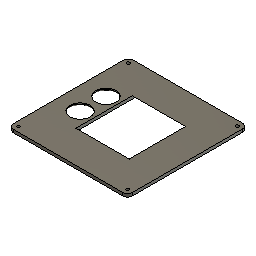
Case_Bottom (Autodesk Fusion 360 design; units mm, degrees)
part number: 2026-02-15-14-31-26-790
Autodesk Fusion 360 part; units mm, degrees
(part 1 of 2)
sketch "Sketch1" plane through (0, 0, 0) normal (0, 1, 0) x (1, 0, 0)
  line L0 (0, 0) -> (98.4, 0)
  line L1 (98.4, 0) -> (98.4, 99.18)
  line L2 (98.4, 99.18) -> (0, 99.18)
  line L3 (0, 99.18) -> (0, 0)
  line L4 (-10, 109.18) -> (108.4, 109.18)
  line L5 (108.4, 109.18) -> (108.4, -10)
  line L6 (108.4, -10) -> (-10, -10)
  line L7 (-10, -10) -> (-10, 109.18)
  circle A0 centre (-5, 104.18) radius 1.45
  circle A1 centre (103.4, 104.18) radius 1.45
  circle A2 centre (-5, -5) radius 1.45
  circle A3 centre (103.4, -5) radius 1.45
  dimension "d1" = 98.4
  dimension "d2" = 99.18
  dimension "d3" = 10
  dimension "d4" = 10
  dimension "d5" = 10
  dimension "d6" = 10
  dimension "d7" = 2.9
  dimension "d8" = 2.9
  dimension "d9" = 2.9
  dimension "d10" = 2.9
  dimension "d11" = 5
  dimension "d12" = 5
  dimension "d13" = 5
  dimension "d14" = 5
  dimension "d15" = 5
  dimension "d16" = 5
  dimension "d17" = 5
  dimension "d18" = 5
  constraint horizontal L0
  constraint vertical L1
  constraint horizontal L2
  constraint vertical L3
  constraint coincident L0.start L3.end
  constraint horizontal L4
  constraint vertical L5
  constraint horizontal L6
  constraint vertical L7
  measures "d1" distance of L0.start L0.end
  measures "d2" distance of L0.start L2.end
  measures "d3" distance of L1 L5
  measures "d4" distance of L3 L7
  measures "d5" distance of L0 L6
  measures "d6" distance of L2 L4
  measures "d7" diameter of A0
  measures "d8" diameter of A1
  measures "d9" diameter of A2
  measures "d10" diameter of A3
  measures "d11" distance of L6 A2.centre
  measures "d12" distance of L7 A2.centre
  measures "d13" distance of L6 A3.centre
  measures "d14" distance of L5 A3.centre
  measures "d15" distance of L4 A1.centre
  measures "d16" distance of L5 A1.centre
  measures "d17" distance of L4 A0.centre
  measures "d18" distance of L7 A0.centre
extrude "Extrude1" add sketch "Sketch1" along normal blind 3 contours L0 L1 L2 L3 | L4 L5 L6 L7 makes body 1
extrude "Extrude2" add sketch "Sketch1" along normal blind 13 bodies 1
sketch "plate-2026-02-16T06_39_50.723Z" plane through (0, 13, 0) normal (0, 1, 0) x (1, 0, 0)
  line L0 (38.525, 61.075) -> (51.525, 61.075)
  line L1 (38.525, 47.075) -> (51.525, 47.075)
  line L2 (38.025, 60.575) -> (38.025, 47.575)
  line L3 (52.025, 60.575) -> (52.025, 47.575)
  arc A0 (38.525, 61.075) -> (38.025, 60.575) centre (38.525, 60.575) ccw
  arc A1 (52.025, 60.575) -> (51.525, 61.075) centre (51.525, 60.575) ccw
  arc A2 (38.025, 47.575) -> (38.525, 47.075) centre (38.525, 47.575) ccw
  arc A3 (51.525, 47.075) -> (52.025, 47.575) centre (51.525, 47.575) ccw
  line L4 (57.575, 61.075) -> (70.575, 61.075)
  line L5 (57.575, 47.075) -> (70.575, 47.075)
  line L6 (57.075, 60.575) -> (57.075, 47.575)
  line L7 (71.075, 60.575) -> (71.075, 47.575)
  arc A4 (57.575, 61.075) -> (57.075, 60.575) centre (57.575, 60.575) ccw
  arc A5 (71.075, 60.575) -> (70.575, 61.075) centre (70.575, 60.575) ccw
  arc A6 (57.075, 47.575) -> (57.575, 47.075) centre (57.575, 47.575) ccw
  arc A7 (70.575, 47.075) -> (71.075, 47.575) centre (70.575, 47.575) ccw
  line L8 (76.625, 61.075) -> (89.625, 61.075)
  line L9 (76.625, 47.075) -> (89.625, 47.075)
  line L10 (76.125, 60.575) -> (76.125, 47.575)
  line L11 (90.125, 60.575) -> (90.125, 47.575)
  arc A8 (76.625, 61.075) -> (76.125, 60.575) centre (76.625, 60.575) ccw
  arc A9 (90.125, 60.575) -> (89.625, 61.075) centre (89.625, 60.575) ccw
  arc A10 (76.125, 47.575) -> (76.625, 47.075) centre (76.625, 47.575) ccw
  arc A11 (89.625, 47.075) -> (90.125, 47.575) centre (89.625, 47.575) ccw
  line L12 (38.525, 42.025) -> (51.525, 42.025)
  line L13 (38.525, 28.025) -> (51.525, 28.025)
  line L14 (38.025, 41.525) -> (38.025, 28.525)
  line L15 (52.025, 41.525) -> (52.025, 28.525)
  arc A12 (38.525, 42.025) -> (38.025, 41.525) centre (38.525, 41.525) ccw
  arc A13 (52.025, 41.525) -> (51.525, 42.025) centre (51.525, 41.525) ccw
  arc A14 (38.025, 28.525) -> (38.525, 28.025) centre (38.525, 28.525) ccw
  arc A15 (51.525, 28.025) -> (52.025, 28.525) centre (51.525, 28.525) ccw
  line L16 (57.575, 42.025) -> (70.575, 42.025)
  line L17 (57.575, 28.025) -> (70.575, 28.025)
  line L18 (57.075, 41.525) -> (57.075, 28.525)
  line L19 (71.075, 41.525) -> (71.075, 28.525)
  arc A16 (57.575, 42.025) -> (57.075, 41.525) centre (57.575, 41.525) ccw
  arc A17 (71.075, 41.525) -> (70.575, 42.025) centre (70.575, 41.525) ccw
  arc A18 (57.075, 28.525) -> (57.575, 28.025) centre (57.575, 28.525) ccw
  arc A19 (70.575, 28.025) -> (71.075, 28.525) centre (70.575, 28.525) ccw
  line L20 (76.625, 42.025) -> (89.625, 42.025)
  line L21 (76.625, 28.025) -> (89.625, 28.025)
  line L22 (76.125, 41.525) -> (76.125, 28.525)
  line L23 (90.125, 41.525) -> (90.125, 28.525)
  arc A20 (76.625, 42.025) -> (76.125, 41.525) centre (76.625, 41.525) ccw
  arc A21 (90.125, 41.525) -> (89.625, 42.025) centre (89.625, 41.525) ccw
  arc A22 (76.125, 28.525) -> (76.625, 28.025) centre (76.625, 28.525) ccw
  arc A23 (89.625, 28.025) -> (90.125, 28.525) centre (89.625, 28.525) ccw
  line L24 (38.525, 22.975) -> (51.525, 22.975)
  line L25 (38.525, 8.975) -> (51.525, 8.975)
  line L26 (38.025, 22.475) -> (38.025, 9.475)
  line L27 (52.025, 22.475) -> (52.025, 9.475)
  arc A24 (38.525, 22.975) -> (38.025, 22.475) centre (38.525, 22.475) ccw
  arc A25 (52.025, 22.475) -> (51.525, 22.975) centre (51.525, 22.475) ccw
  arc A26 (38.025, 9.475) -> (38.525, 8.975) centre (38.525, 9.475) ccw
  arc A27 (51.525, 8.975) -> (52.025, 9.475) centre (51.525, 9.475) ccw
  line L28 (57.575, 22.975) -> (70.575, 22.975)
  line L29 (57.575, 8.975) -> (70.575, 8.975)
  line L30 (57.075, 22.475) -> (57.075, 9.475)
  line L31 (71.075, 22.475) -> (71.075, 9.475)
  arc A28 (57.575, 22.975) -> (57.075, 22.475) centre (57.575, 22.475) ccw
  arc A29 (71.075, 22.475) -> (70.575, 22.975) centre (70.575, 22.475) ccw
  arc A30 (57.075, 9.475) -> (57.575, 8.975) centre (57.575, 9.475) ccw
  arc A31 (70.575, 8.975) -> (71.075, 9.475) centre (70.575, 9.475) ccw
  line L32 (76.625, 22.975) -> (89.625, 22.975)
  line L33 (76.625, 8.975) -> (89.625, 8.975)
  line L34 (76.125, 22.475) -> (76.125, 9.475)
  line L35 (90.125, 22.475) -> (90.125, 9.475)
  arc A32 (76.625, 22.975) -> (76.125, 22.475) centre (76.625, 22.475) ccw
  arc A33 (90.125, 22.475) -> (89.625, 22.975) centre (89.625, 22.475) ccw
  arc A34 (76.125, 9.475) -> (76.625, 8.975) centre (76.625, 9.475) ccw
  arc A35 (89.625, 8.975) -> (90.125, 9.475) centre (89.625, 9.475) ccw
  line L36 (35.5, 6.45) -> (92.65, 6.45)
  line L37 (35.5, 63.6) -> (92.65, 63.6)
  line L38 (35.5, 6.45) -> (35.5, 63.6)
  line L39 (92.65, 6.45) -> (92.65, 63.6)
sketch "Sketch3" plane through (0, 13, 0) normal (0, 1, 0) x (-1, 0, 0)
  line L0 (0, 0) -> (0, -99.18)
  line L1 (0, -99.18) -> (-98.4, -99.18)
  line L2 (-98.4, -99.18) -> (-98.4, 0)
  line L3 (-98.4, 0) -> (0, 0)
  circle A0 centre (5, -104.18) radius 1.45
  circle A1 centre (5, 5) radius 1.45
  circle A2 centre (-103.4, -104.18) radius 1.45
  circle A3 centre (-103.4, 5) radius 1.45
  line L4 (10, 10) -> (-108.4, 10)
  line L5 (-108.4, 10) -> (-108.4, -109.18)
  line L6 (-108.4, -109.18) -> (10, -109.18)
  line L7 (10, -109.18) -> (10, 10)
  line L8 (-98.4, 0) -> (0, 0)
  line L9 (0, 0) -> (0, -99.18)
  line L10 (0, -99.18) -> (-98.4, -99.18)
  line L11 (-98.4, -99.18) -> (-98.4, 0)
  constraint horizontal L8
  constraint vertical L9
  constraint horizontal L10
  constraint vertical L11
  constraint coincident L0.end L1.start
  constraint coincident L2.end L3.start
sketch "plate-2026-02-16T06_39_50.723Z (1)" plane through (0, 13, 0) normal (0, 1, 0) x (1, 0, 0)
  line L0 (38.525, 61.075) -> (51.525, 61.075)
  line L1 (38.525, 47.075) -> (51.525, 47.075)
  line L2 (38.025, 60.575) -> (38.025, 47.575)
  line L3 (52.025, 60.575) -> (52.025, 47.575)
  arc A0 (38.525, 61.075) -> (38.025, 60.575) centre (38.525, 60.575) ccw
  arc A1 (52.025, 60.575) -> (51.525, 61.075) centre (51.525, 60.575) ccw
  arc A2 (38.025, 47.575) -> (38.525, 47.075) centre (38.525, 47.575) ccw
  arc A3 (51.525, 47.075) -> (52.025, 47.575) centre (51.525, 47.575) ccw
  line L4 (57.575, 61.075) -> (70.575, 61.075)
  line L5 (57.575, 47.075) -> (70.575, 47.075)
  line L6 (57.075, 60.575) -> (57.075, 47.575)
  line L7 (71.075, 60.575) -> (71.075, 47.575)
  arc A4 (57.575, 61.075) -> (57.075, 60.575) centre (57.575, 60.575) ccw
  arc A5 (71.075, 60.575) -> (70.575, 61.075) centre (70.575, 60.575) ccw
  arc A6 (57.075, 47.575) -> (57.575, 47.075) centre (57.575, 47.575) ccw
  arc A7 (70.575, 47.075) -> (71.075, 47.575) centre (70.575, 47.575) ccw
  line L8 (76.625, 61.075) -> (89.625, 61.075)
  line L9 (76.625, 47.075) -> (89.625, 47.075)
  line L10 (76.125, 60.575) -> (76.125, 47.575)
  line L11 (90.125, 60.575) -> (90.125, 47.575)
  arc A8 (76.625, 61.075) -> (76.125, 60.575) centre (76.625, 60.575) ccw
  arc A9 (90.125, 60.575) -> (89.625, 61.075) centre (89.625, 60.575) ccw
  arc A10 (76.125, 47.575) -> (76.625, 47.075) centre (76.625, 47.575) ccw
  arc A11 (89.625, 47.075) -> (90.125, 47.575) centre (89.625, 47.575) ccw
  line L12 (38.525, 42.025) -> (51.525, 42.025)
  line L13 (38.525, 28.025) -> (51.525, 28.025)
  line L14 (38.025, 41.525) -> (38.025, 28.525)
  line L15 (52.025, 41.525) -> (52.025, 28.525)
  arc A12 (38.525, 42.025) -> (38.025, 41.525) centre (38.525, 41.525) ccw
  arc A13 (52.025, 41.525) -> (51.525, 42.025) centre (51.525, 41.525) ccw
  arc A14 (38.025, 28.525) -> (38.525, 28.025) centre (38.525, 28.525) ccw
  arc A15 (51.525, 28.025) -> (52.025, 28.525) centre (51.525, 28.525) ccw
  line L16 (57.575, 42.025) -> (70.575, 42.025)
  line L17 (57.575, 28.025) -> (70.575, 28.025)
  line L18 (57.075, 41.525) -> (57.075, 28.525)
  line L19 (71.075, 41.525) -> (71.075, 28.525)
  arc A16 (57.575, 42.025) -> (57.075, 41.525) centre (57.575, 41.525) ccw
  arc A17 (71.075, 41.525) -> (70.575, 42.025) centre (70.575, 41.525) ccw
  arc A18 (57.075, 28.525) -> (57.575, 28.025) centre (57.575, 28.525) ccw
  arc A19 (70.575, 28.025) -> (71.075, 28.525) centre (70.575, 28.525) ccw
  line L20 (76.625, 42.025) -> (89.625, 42.025)
  line L21 (76.625, 28.025) -> (89.625, 28.025)
  line L22 (76.125, 41.525) -> (76.125, 28.525)
  line L23 (90.125, 41.525) -> (90.125, 28.525)
  arc A20 (76.625, 42.025) -> (76.125, 41.525) centre (76.625, 41.525) ccw
  arc A21 (90.125, 41.525) -> (89.625, 42.025) centre (89.625, 41.525) ccw
  arc A22 (76.125, 28.525) -> (76.625, 28.025) centre (76.625, 28.525) ccw
  arc A23 (89.625, 28.025) -> (90.125, 28.525) centre (89.625, 28.525) ccw
  line L24 (38.525, 22.975) -> (51.525, 22.975)
  line L25 (38.525, 8.975) -> (51.525, 8.975)
  line L26 (38.025, 22.475) -> (38.025, 9.475)
  line L27 (52.025, 22.475) -> (52.025, 9.475)
  arc A24 (38.525, 22.975) -> (38.025, 22.475) centre (38.525, 22.475) ccw
  arc A25 (52.025, 22.475) -> (51.525, 22.975) centre (51.525, 22.475) ccw
  arc A26 (38.025, 9.475) -> (38.525, 8.975) centre (38.525, 9.475) ccw
  arc A27 (51.525, 8.975) -> (52.025, 9.475) centre (51.525, 9.475) ccw
  line L28 (57.575, 22.975) -> (70.575, 22.975)
  line L29 (57.575, 8.975) -> (70.575, 8.975)
  line L30 (57.075, 22.475) -> (57.075, 9.475)
  line L31 (71.075, 22.475) -> (71.075, 9.475)
  arc A28 (57.575, 22.975) -> (57.075, 22.475) centre (57.575, 22.475) ccw
  arc A29 (71.075, 22.475) -> (70.575, 22.975) centre (70.575, 22.475) ccw
  arc A30 (57.075, 9.475) -> (57.575, 8.975) centre (57.575, 9.475) ccw
  arc A31 (70.575, 8.975) -> (71.075, 9.475) centre (70.575, 9.475) ccw
  line L32 (76.625, 22.975) -> (89.625, 22.975)
  line L33 (76.625, 8.975) -> (89.625, 8.975)
  line L34 (76.125, 22.475) -> (76.125, 9.475)
  line L35 (90.125, 22.475) -> (90.125, 9.475)
  arc A32 (76.625, 22.975) -> (76.125, 22.475) centre (76.625, 22.475) ccw
  arc A33 (90.125, 22.475) -> (89.625, 22.975) centre (89.625, 22.475) ccw
  arc A34 (76.125, 9.475) -> (76.625, 8.975) centre (76.625, 9.475) ccw
  arc A35 (89.625, 8.975) -> (90.125, 9.475) centre (89.625, 9.475) ccw
  line L36 (35.5, 6.45) -> (92.65, 6.45)
  line L37 (35.5, 63.6) -> (92.65, 63.6)
  line L38 (35.5, 6.45) -> (35.5, 63.6)
  line L39 (92.65, 6.45) -> (92.65, 63.6)
  line L40 (98.4, 99.18) -> (98.4, 0)
  dimension "d137" = 5.75
  measures "d137" distance of L39 L40
extrude "Extrude3" add sketch "Sketch3" along normal blind 3 separate body contours L0 L1 L2 L3 L8 L9 L10 L11 | L4 L5 L6 L7 makes body 2
extrude "Extrude4" add sketch "plate-2026-02-16T06_39_50.723Z" sketch "plate-2026-02-16T06_39_50.723Z (1)" along normal blind 3 contours L0 L1 L2 L3 A0 A1 A2 A3 | L20 L21 L22 L23 A20 A21 A22 A23 | L24 L25 L26 L27 A24 A25 A26 A27 | L32 L33 L34 L35 A32 A33 A34 A35 of sketch 2 contours L4 L5 L6 L7 A4 A5 A6 A7 | L8 L9 L10 L11 A8 A9 A10 A11 | L12 L13 L14 L15 A12 A13 A14 A15 | L16 L17 L18 L19 A16 A17 A18 A19 | L28 L29 L30 L31 A28 A29 A30 A31 bodies 2
sketch "Sketch5" plane through (0, 16, 0) normal (0, 1, 0) x (-1, 0, 0)
  circle A0 centre (5, 5) radius 1.45
  circle A1 centre (5, -104.18) radius 1.45
  circle A2 centre (-103.4, 5) radius 1.45
  circle A3 centre (-103.4, -104.18) radius 1.45
  line L0 (10, -109.18) -> (10, 10)
  line L1 (10, 10) -> (-108.4, 10)
  line L2 (-108.4, 10) -> (-108.4, -109.18)
  line L3 (-108.4, -109.18) -> (10, -109.18)
  line L4 (-37.72, -73.425) -> (-67.22, -73.425)
  line L5 (-67.22, -73.425) -> (-67.22, -85.425)
  line L6 (-67.22, -85.425) -> (-37.72, -85.425)
  line L7 (-37.72, -85.425) -> (-37.72, -73.425)
  line L8 (-98.4, 0, -16) -> (-98.4, -99.18, -16)
  line L9 (-98.4, -80.7281, -16) -> (-98.4, -78.7, -16)
  line L10 (-93.6, -70.6895, -3) -> (-93.6, -82.5535, -3)
  line L11 (-93.6, -99.18, -3) -> (-93.6, 0, -3)
  dimension "d27" = 29.5
  dimension "d28" = 12
  constraint horizontal L4
  constraint vertical L5
  constraint horizontal L6
  constraint vertical L7
  measures "d27" distance of L4.start L4.end
  measures "d28" distance of L4.start L6.end
extrude "Extrude5" cut sketch "Sketch5" against normal blind 3 contours L4 L5 L6 L7 bodies 2 1
sketch "Sketch6" plane through (0, 16, 0) normal (0, 1, 0) x (-1, 0, 0)
  line L0 (-67.22, -73.425) -> (-37.72, -73.425)
  line L1 (-37.72, -73.425) -> (-37.72, -85.425)
  line L2 (-37.72, -85.425) -> (-67.22, -85.425)
  line L3 (-67.22, -85.425) -> (-67.22, -73.425)
  circle A0 centre (5, 5) radius 1.45
  circle A1 centre (5, -104.18) radius 1.45
  circle A2 centre (-103.4, 5) radius 1.45
  circle A3 centre (-103.4, -104.18) radius 1.45
  line L4 (10, -109.18) -> (10, 10)
  line L5 (10, 10) -> (-108.4, 10)
  line L6 (-108.4, 10) -> (-108.4, -109.18)
  line L7 (-108.4, -109.18) -> (10, -109.18)
  line L8 (-0.6538, -95.1906, -15.0539) -> (-36.0838, -95.1906, -15.0539)
  line L9 (-36.0838, -95.1906, -15.0539) -> (-36.0838, -10.4306, -15.0539)
  line L10 (-36.0838, -10.4306, -15.0539) -> (-0.6538, -10.4306, -15.0539)
  line L11 (-0.6538, -10.4306, -15.0539) -> (-0.6538, -95.1906, -15.0539)
  line L12 (0, 0, -16) -> (-98.4, 0, -16)
  line L13 (-98.4, -99.18, -16) -> (0, -99.18, -16)
  line L14 (0, -99.18, -16) -> (0, 0, -16)
  dimension "d32" = 35.43
  dimension "d33" = 84.76
  dimension "d35" = 4.1
  dimension "d36" = 1.15
extrude "Extrude6" cut sketch "Sketch6" along normal blind 30 contours L8 L9 L10 L11 in plane through (0, 0.9461, 0) normal (0, 1, 0) bodies 1 2
move_face "MoveFace1" by (0, 2, 0) 1 faces at (12.4638, 0.9461, -38.684) on bodies 1
sketch "Sketch7" plane through (108.4, 0, 0) normal (1, 0, 0) x (0, 0, -1)
  line L0 (-10, 0) -> (109.18, 0)
  line L1 (109.18, 13) -> (109.18, 16)
  line L2 (109.18, 16) -> (-10, 16)
  line L3 (-10, 16) -> (-10, 13)
  line L4 (81.805, 13, -10) -> (95.805, 13, -10)
  line L5 (95.805, 13, -10) -> (95.805, 8.2, -10)
  line L6 (95.805, 8.2, -10) -> (81.805, 8.2, -10)
  line L7 (81.805, 8.2, -10) -> (81.805, 13, -10)
  line L8 (99.18, 13, -10) -> (0, 13, -10)
  line L9 (-10, 13) -> (109.18, 13)
  line L10 (109.18, 0) -> (109.18, 13)
  line L11 (109.18, 13) -> (-10, 13)
  line L12 (-10, 13) -> (-10, 0)
  line L13 (78.48, 5) -> (92.48, 5)
  line L14 (92.48, 5) -> (92.48, 13)
  line L15 (92.48, 13) -> (78.48, 13)
  line L16 (78.48, 13) -> (78.48, 5)
  dimension "d42" = 14
  dimension "d43" = 16.7
  dimension "d62" = 4.8
  dimension "d64" = 16.7
  dimension "d65" = 0
  constraint horizontal L13
  constraint vertical L14
  constraint horizontal L15
  constraint vertical L16
  measures "d64" distance of L10 L14
  measures "d65" distance of L16
extrude "Extrude7" cut sketch "Sketch7" against normal blind 10 contours L9 L11 L13 L14 L15 L16 bodies 1
fillet "Fillet1" radius 5 1 edges at (36.0838, 14.5, -95.1906) on bodies 2
fillet "Fillet2" radius 5 1 edges at (0.6538, 14.5, -95.1906) on bodies 2
fillet "Fillet3" radius 5 1 edges at (36.0838, 14.5, -10.4306) on bodies 2
fillet "Fillet4" radius 5 1 edges at (0.6538, 14.5, -10.4306) on bodies 2
fillet "Fillet5" radius 2 1 edges at (37.72, 14.5, -85.425) on bodies 2
fillet "Fillet6" radius 2 1 edges at (67.22, 14.5, -85.425) on bodies 2
fillet "Fillet7" radius 2 1 edges at (67.22, 14.5, -73.425) on bodies 2
fillet "Fillet8" radius 2 1 edges at (37.72, 14.5, -73.425) on bodies 2
fillet "Fillet9" radius 2 1 edges at (103.4, 5, -92.48) on bodies 1
fillet "Fillet10" radius 2 1 edges at (103.4, 5, -78.48) on bodies 1
fillet "Fillet11" radius 5 1 edges at (108.4, 6.5, -109.18) on bodies 1
fillet "Fillet12" radius 5 1 edges at (108.4, 14.5, -109.18) on bodies 2
fillet "Fillet13" radius 5 1 edges at (-10, 6.5, -109.18) on bodies 1
fillet "Fillet14" radius 5 1 edges at (-10, 14.5, -109.18) on bodies 2
fillet "Fillet15" radius 5 2 edges at (-10, 6.5, 10) (-10, 14.5, 10) on bodies 1 2
fillet "Fillet16" radius 5 2 edges at (108.4, 6.5, 10) (108.4, 14.5, 10) on bodies 1 2
sketch "Sketch8" plane through (0, 16, 0) normal (0, 1, 0) x (-1, 0, 0)
  arc A0 (-103.4, 10) -> (-108.4, 5) centre (-103.4, 5) ccw
  line L0 (-108.4, 5) -> (-108.4, -104.18)
  arc A1 (-108.4, -104.18) -> (-103.4, -109.18) centre (-103.4, -104.18) ccw
  line L1 (-103.4, -109.18) -> (5, -109.18)
  arc A2 (5, -109.18) -> (10, -104.18) centre (5, -104.18) ccw
  line L2 (10, -104.18) -> (10, 5)
  arc A3 (10, 5) -> (5, 10) centre (5, 5) ccw
  line L3 (5, 10) -> (-103.4, 10)
  line L4 (-0.6538, -15.4306) -> (-0.6538, -90.1906)
  arc A4 (-5.6538, -95.1906) -> (-0.6538, -90.1906) centre (-5.6538, -90.1906) ccw
  line L5 (-5.6538, -95.1906) -> (-31.0838, -95.1906)
  arc A5 (-36.0838, -90.1906) -> (-31.0838, -95.1906) centre (-31.0838, -90.1906) ccw
  line L6 (-36.0838, -90.1906) -> (-36.0838, -15.4306)
  arc A6 (-31.0838, -10.4306) -> (-36.0838, -15.4306) centre (-31.0838, -15.4306) ccw
  line L7 (-31.0838, -10.4306) -> (-5.6538, -10.4306)
  arc A7 (-0.6538, -15.4306) -> (-5.6538, -10.4306) centre (-5.6538, -15.4306) ccw
  line L8 (-65.22, -73.425) -> (-39.72, -73.425)
  arc A8 (-37.72, -75.425) -> (-39.72, -73.425) centre (-39.72, -75.425) ccw
  line L9 (-37.72, -75.425) -> (-37.72, -83.425)
  arc A9 (-39.72, -85.425) -> (-37.72, -83.425) centre (-39.72, -83.425) ccw
  line L10 (-39.72, -85.425) -> (-65.22, -85.425)
  arc A10 (-67.22, -83.425) -> (-65.22, -85.425) centre (-65.22, -83.425) ccw
  line L11 (-67.22, -83.425) -> (-67.22, -75.425)
  arc A11 (-65.22, -73.425) -> (-67.22, -75.425) centre (-65.22, -75.425) ccw
  circle A12 centre (-103.4, 5) radius 1.45
  circle A13 centre (-103.4, -104.18) radius 1.45
  circle A14 centre (5, 5) radius 1.45
  circle A15 centre (5, -104.18) radius 1.45
  line L12 (-75, -95) -> (-75, -73.1115)
  line L13 (-75, -73.1115) -> (-75, -95)
  line L14 (-75, -95) -> (-96.8748, -95)
  line L15 (-77, -75) -> (-77, -93)
  line L16 (-77, -93) -> (-95, -93)
  line L17 (-79, -77) -> (-79, -91)
  line L18 (-79, -91) -> (-93, -91)
  line L19 (-81, -79) -> (-81, -89)
  line L20 (-81, -89) -> (-91, -89)
  line L21 (-75, -73.1115) -> (-77, -75)
  line L22 (-79, -77) -> (-81, -79)
  line L23 (-96.8748, -95) -> (-95, -93)
  line L24 (-93, -91) -> (-91, -89)
  line L25 (-83, -81) -> (-83, -87)
  line L26 (-83, -87) -> (-89, -87)
  line L27 (-85, -83) -> (-85, -85.23)
  line L28 (-85, -85.23) -> (-87, -85.23)
  line L29 (-87, -85.23) -> (-89, -87)
  line L30 (-85, -83) -> (-83, -81)
  line L31 (-73, -68) -> (-102, -97)
  line L32 (-100, -70) -> (-100, -91.8748)
  line L33 (-98, -72) -> (-98, -90)
  line L34 (-96, -74) -> (-96, -88)
  line L35 (-94, -76) -> (-94, -86)
  line L36 (-92, -78) -> (-92, -84)
  line L37 (-90.23, -80) -> (-90.23, -82)
  line L38 (-90.23, -82) -> (-92, -84)
  line L39 (-96, -88) -> (-94, -86)
  line L40 (-100, -91.8748) -> (-98, -90)
  line L41 (-100, -70) -> (-78.1115, -70)
  line L42 (-80, -72) -> (-98, -72)
  line L43 (-82, -74) -> (-96, -74)
  line L44 (-84, -76) -> (-94, -76)
  line L45 (-86, -78) -> (-92, -78)
  line L46 (-88, -80) -> (-86, -78)
  line L47 (-88, -80) -> (-90.23, -80)
  line L48 (-82, -74) -> (-84, -76)
  line L49 (-78.1115, -70) -> (-80, -72)
  constraint vertical L12
  constraint perpendicular L13 L14
  constraint parallel L13 L15
  constraint perpendicular L15 L16
  constraint vertical L17
  constraint perpendicular L17 L18
  constraint vertical L19
  constraint perpendicular L19 L20
  constraint vertical L25
  constraint perpendicular L25 L26
  constraint parallel L25 L27
  constraint perpendicular L25 L28
  constraint symmetric L12.start L31 L32.start
  constraint symmetric L12.end L31 L41.end
  constraint symmetric L14.end L31 L32.end
  constraint symmetric L15.start L31 L42.start
  constraint symmetric L15.end L31 L33.start
  constraint symmetric L16.end L31 L33.end
  constraint symmetric L17.start L31 L43.start
  constraint symmetric L17.end L31 L34.start
  constraint symmetric L18.end L31 L34.end
  constraint symmetric L19.start L31 L44.start
  constraint symmetric L19.end L31 L35.start
  constraint symmetric L20.end L31 L35.end
  constraint symmetric L25.start L31 L45.start
  constraint symmetric L25.end L31 L36.start
  constraint symmetric L26.end L31 L36.end
  constraint symmetric L27.start L31 L46.start
  constraint symmetric L27.end L31 L37.start
  constraint symmetric L28.end L31 L37.end
extrude "Extrude8" cut sketch "Sketch8" against normal blind 3 contours L12 L13 L14 L15 L16 L21 L23 | L17 L18 L19 L20 L22 L24 | L25 L26 L27 L28 L29 L30 | L32 L33 L40 L41 L42 L49 | L34 L35 L39 L43 L44 L48 | L36 L37 L38 L45 L46 L47 bodies 2
sketch "Sketch9" plane through (0, 16, 0) normal (0, 1, 0) x (-1, 0, 0)
  line L0 (-89, -87) -> (-87, -85.23)
  line L1 (-87, -85.23) -> (-85, -85.23)
  line L2 (-85, -85.23) -> (-85, -83)
  line L3 (-85, -83) -> (-83, -81)
  line L4 (-83, -81) -> (-83, -87)
  line L5 (-83, -87) -> (-89, -87)
  line L6 (-98, -90) -> (-100, -91.8748)
  line L7 (-100, -91.8748) -> (-100, -70)
  line L8 (-100, -70) -> (-78.1115, -70)
  line L9 (-78.1115, -70) -> (-80, -72)
  line L10 (-80, -72) -> (-98, -72)
  line L11 (-98, -72) -> (-98, -90)
  line L12 (-81, -89) -> (-81, -79)
  line L13 (-81, -79) -> (-79, -77)
  line L14 (-79, -77) -> (-79, -91)
  line L15 (-79, -91) -> (-93, -91)
  line L16 (-93, -91) -> (-91, -89)
  line L17 (-91, -89) -> (-81, -89)
  line L18 (-92, -84) -> (-92, -78)
  line L19 (-92, -78) -> (-86, -78)
  line L20 (-86, -78) -> (-88, -80)
  line L21 (-88, -80) -> (-90.23, -80)
  line L22 (-90.23, -80) -> (-90.23, -82)
  line L23 (-90.23, -82) -> (-92, -84)
  line L24 (-94, -86) -> (-96, -88)
  line L25 (-96, -88) -> (-96, -74)
  line L26 (-96, -74) -> (-82, -74)
  line L27 (-82, -74) -> (-84, -76)
  line L28 (-84, -76) -> (-94, -76)
  line L29 (-94, -76) -> (-94, -86)
  line L30 (-77, -93) -> (-77, -75)
  line L31 (-77, -75) -> (-75, -73.1115)
  line L32 (-75, -73.1115) -> (-75, -95)
  line L33 (-75, -95) -> (-96.8748, -95)
  line L34 (-96.8748, -95) -> (-95, -93)
  line L35 (-95, -93) -> (-77, -93)
  arc A0 (-103.4, 10) -> (-108.4, 5) centre (-103.4, 5) ccw
  line L36 (-108.4, 5) -> (-108.4, -104.18)
  arc A1 (-108.4, -104.18) -> (-103.4, -109.18) centre (-103.4, -104.18) ccw
  line L37 (-103.4, -109.18) -> (5, -109.18)
  arc A2 (5, -109.18) -> (10, -104.18) centre (5, -104.18) ccw
  line L38 (10, -104.18) -> (10, 5)
  arc A3 (10, 5) -> (5, 10) centre (5, 5) ccw
  line L39 (5, 10) -> (-103.4, 10)
  line L40 (-0.6538, -15.4306) -> (-0.6538, -90.1906)
  arc A4 (-5.6538, -95.1906) -> (-0.6538, -90.1906) centre (-5.6538, -90.1906) ccw
  line L41 (-5.6538, -95.1906) -> (-31.0838, -95.1906)
  arc A5 (-36.0838, -90.1906) -> (-31.0838, -95.1906) centre (-31.0838, -90.1906) ccw
  line L42 (-36.0838, -90.1906) -> (-36.0838, -15.4306)
  arc A6 (-31.0838, -10.4306) -> (-36.0838, -15.4306) centre (-31.0838, -15.4306) ccw
  line L43 (-31.0838, -10.4306) -> (-5.6538, -10.4306)
  arc A7 (-0.6538, -15.4306) -> (-5.6538, -10.4306) centre (-5.6538, -15.4306) ccw
  line L44 (-65.22, -73.425) -> (-39.72, -73.425)
  arc A8 (-37.72, -75.425) -> (-39.72, -73.425) centre (-39.72, -75.425) ccw
  line L45 (-37.72, -75.425) -> (-37.72, -83.425)
  arc A9 (-39.72, -85.425) -> (-37.72, -83.425) centre (-39.72, -83.425) ccw
  line L46 (-39.72, -85.425) -> (-65.22, -85.425)
  arc A10 (-67.22, -83.425) -> (-65.22, -85.425) centre (-65.22, -83.425) ccw
  line L47 (-67.22, -83.425) -> (-67.22, -75.425)
  arc A11 (-65.22, -73.425) -> (-67.22, -75.425) centre (-65.22, -75.425) ccw
  circle A12 centre (-103.4, 5) radius 1.45
  circle A13 centre (-103.4, -104.18) radius 1.45
  circle A14 centre (5, 5) radius 1.45
  circle A15 centre (5, -104.18) radius 1.45
  line L48 (0, -5) -> (-90, -5)
  line L49 (-90, -5) -> (-90, 0)
  line L50 (-90, 0) -> (0, 0)
  line L51 (0, 0) -> (0, -5)
  line L52 (0, -5) -> (-5, 0)
  line L53 (-5, -5) -> (-10, 0)
  line L54 (-10, -5) -> (-15, 0)
  line L55 (-15, -5) -> (-20, 0)
  line L56 (-20, -5) -> (-25, 0)
  line L57 (-25, -5) -> (-30, 0)
  line L58 (-30, -5) -> (-35, 0)
  line L59 (-35, -5) -> (-40, 0)
  line L60 (-40, -5) -> (-45, 0)
  line L61 (-45, -5) -> (-50, 0)
  line L62 (-50, -5) -> (-55, 0)
  line L63 (-55, -5) -> (-60, 0)
  line L64 (-60, -5) -> (-65, 0)
  line L65 (-65, -5) -> (-70, 0)
  line L66 (-70, -5) -> (-75, 0)
  line L67 (-75, -5) -> (-80, 0)
  line L68 (-80, -5) -> (-85, 0)
  line L69 (-85, -5) -> (-90, 0)
  line L70 (-85.1002, -5) -> (-90, 0)
  constraint horizontal L48
  constraint vertical L49
  constraint horizontal L50
  constraint vertical L51
  constraint coincident L50 L52.end
  constraint coincident L48 L53.start
  constraint coincident L50 L53.end
  constraint parallel L52 L53
  constraint coincident L48 L54.start
  constraint coincident L50 L54.end
  constraint parallel L53 L54
  constraint coincident L48 L55.start
  constraint coincident L50 L55.end
  constraint parallel L54 L55
  constraint coincident L48 L56.start
  constraint coincident L50 L56.end
  constraint parallel L55 L56
  constraint coincident L48 L57.start
  constraint coincident L50 L57.end
  constraint parallel L56 L57
  constraint coincident L48 L58.start
  constraint coincident L50 L58.end
  constraint parallel L57 L58
  constraint coincident L48 L59.start
  constraint coincident L50 L59.end
  constraint parallel L58 L59
  constraint coincident L48 L60.start
  constraint coincident L50 L60.end
  constraint parallel L59 L60
  constraint coincident L48 L61.start
  constraint coincident L50 L61.end
  constraint parallel L60 L61
  constraint coincident L48 L62.start
  constraint coincident L50 L62.end
  constraint parallel L61 L62
  constraint coincident L48 L63.start
  constraint coincident L50 L63.end
  constraint parallel L62 L63
  constraint coincident L48 L64.start
  constraint coincident L50 L64.end
  constraint parallel L62 L64
  constraint coincident L48 L65.start
  constraint coincident L50 L65.end
  constraint parallel L64 L65
  constraint coincident L48 L66.start
  constraint coincident L50 L66.end
  constraint parallel L65 L66
  constraint coincident L48 L67.start
  constraint coincident L50 L67.end
  constraint parallel L66 L67
  constraint coincident L48 L68.start
  constraint coincident L50 L68.end
  constraint parallel L67 L68
  constraint coincident L48 L69.start
  constraint coincident L50 L49.end
  constraint parallel L68 L69
  constraint coincident L48 L70.start
extrude "Extrude9" cut sketch "Sketch9" against normal blind 5 contours L50 L51 L52 | L48 L50 L53 L54 | L48 L50 L55 L56 | L48 L50 L57 L58 | L48 L50 L59 L60 | L48 L50 L61 L62 | L48 L50 L63 L64 | L48 L50 L65 L66 | L48 L50 L67 L68 | L48 L49 L70 bodies 2
sketch "Sketch10" plane through (0, 16, 0) normal (0, 1, 0) x (-1, 0, 0)
  line L0 (-75, 0) -> (-70, 0)
  line L1 (-70, 0) -> (-65, -5)
  line L2 (-65, -5) -> (-70, -5)
  line L3 (-70, -5) -> (-75, 0)
  line L4 (-35, 0) -> (-30, 0)
  line L5 (-30, 0) -> (-25, -5)
  line L6 (-25, -5) -> (-30, -5)
  line L7 (-30, -5) -> (-35, 0)
  line L8 (-5, 0) -> (0, 0)
  line L9 (0, 0) -> (0, -5)
  line L10 (0, -5) -> (-5, 0)
  line L11 (-45, 0) -> (-40, 0)
  line L12 (-40, 0) -> (-35, -5)
  line L13 (-35, -5) -> (-40, -5)
  line L14 (-40, -5) -> (-45, 0)
  line L15 (-85, 0) -> (-80, 0)
  line L16 (-80, 0) -> (-75, -5)
  line L17 (-75, -5) -> (-80, -5)
  line L18 (-80, -5) -> (-85, 0)
  line L19 (-65, 0) -> (-60, 0)
  line L20 (-60, 0) -> (-55, -5)
  line L21 (-55, -5) -> (-60, -5)
  line L22 (-60, -5) -> (-65, 0)
  line L23 (-25, 0) -> (-20, 0)
  line L24 (-20, 0) -> (-15, -5)
  line L25 (-15, -5) -> (-20, -5)
  line L26 (-20, -5) -> (-25, 0)
  line L27 (-15, 0) -> (-10, 0)
  line L28 (-10, 0) -> (-5, -5)
  line L29 (-5, -5) -> (-10, -5)
  line L30 (-10, -5) -> (-15, 0)
  line L31 (-55, 0) -> (-50, 0)
  line L32 (-50, 0) -> (-45, -5)
  line L33 (-45, -5) -> (-50, -5)
  line L34 (-50, -5) -> (-55, 0)
  line L35 (-90, 0) -> (-85.1002, -5)
  line L36 (-85.1002, -5) -> (-90, -5)
  line L37 (-90, -5) -> (-90, 0)
  line L38 (-89, -87) -> (-87, -85.23)
  line L39 (-87, -85.23) -> (-85, -85.23)
  line L40 (-85, -85.23) -> (-85, -83)
  line L41 (-85, -83) -> (-83, -81)
  line L42 (-83, -81) -> (-83, -87)
  line L43 (-83, -87) -> (-89, -87)
  line L44 (-98, -90) -> (-100, -91.8748)
  line L45 (-100, -91.8748) -> (-100, -70)
  line L46 (-100, -70) -> (-78.1115, -70)
  line L47 (-78.1115, -70) -> (-80, -72)
  line L48 (-80, -72) -> (-98, -72)
  line L49 (-98, -72) -> (-98, -90)
  line L50 (-81, -89) -> (-81, -79)
  line L51 (-81, -79) -> (-79, -77)
  line L52 (-79, -77) -> (-79, -91)
  line L53 (-79, -91) -> (-93, -91)
  line L54 (-93, -91) -> (-91, -89)
  line L55 (-91, -89) -> (-81, -89)
  line L56 (-92, -84) -> (-92, -78)
  line L57 (-92, -78) -> (-86, -78)
  line L58 (-86, -78) -> (-88, -80)
  line L59 (-88, -80) -> (-90.23, -80)
  line L60 (-90.23, -80) -> (-90.23, -82)
  line L61 (-90.23, -82) -> (-92, -84)
  line L62 (-94, -86) -> (-96, -88)
  line L63 (-96, -88) -> (-96, -74)
  line L64 (-96, -74) -> (-82, -74)
  line L65 (-82, -74) -> (-84, -76)
  line L66 (-84, -76) -> (-94, -76)
  line L67 (-94, -76) -> (-94, -86)
  line L68 (-77, -93) -> (-77, -75)
  line L69 (-77, -75) -> (-75, -73.1115)
  line L70 (-75, -73.1115) -> (-75, -95)
  line L71 (-75, -95) -> (-96.8748, -95)
  line L72 (-96.8748, -95) -> (-95, -93)
  line L73 (-95, -93) -> (-77, -93)
  arc A0 (-103.4, 10) -> (-108.4, 5) centre (-103.4, 5) ccw
  line L74 (-108.4, 5) -> (-108.4, -104.18)
  arc A1 (-108.4, -104.18) -> (-103.4, -109.18) centre (-103.4, -104.18) ccw
  line L75 (-103.4, -109.18) -> (5, -109.18)
  arc A2 (5, -109.18) -> (10, -104.18) centre (5, -104.18) ccw
  line L76 (10, -104.18) -> (10, 5)
  arc A3 (10, 5) -> (5, 10) centre (5, 5) ccw
  line L77 (5, 10) -> (-103.4, 10)
  line L78 (-0.6538, -15.4306) -> (-0.6538, -90.1906)
  arc A4 (-5.6538, -95.1906) -> (-0.6538, -90.1906) centre (-5.6538, -90.1906) ccw
  line L79 (-5.6538, -95.1906) -> (-31.0838, -95.1906)
  arc A5 (-36.0838, -90.1906) -> (-31.0838, -95.1906) centre (-31.0838, -90.1906) ccw
  line L80 (-36.0838, -90.1906) -> (-36.0838, -15.4306)
  arc A6 (-31.0838, -10.4306) -> (-36.0838, -15.4306) centre (-31.0838, -15.4306) ccw
  line L81 (-31.0838, -10.4306) -> (-5.6538, -10.4306)
  arc A7 (-0.6538, -15.4306) -> (-5.6538, -10.4306) centre (-5.6538, -15.4306) ccw
  line L82 (-65.22, -73.425) -> (-39.72, -73.425)
  arc A8 (-37.72, -75.425) -> (-39.72, -73.425) centre (-39.72, -75.425) ccw
  line L83 (-37.72, -75.425) -> (-37.72, -83.425)
  arc A9 (-39.72, -85.425) -> (-37.72, -83.425) centre (-39.72, -83.425) ccw
  line L84 (-39.72, -85.425) -> (-65.22, -85.425)
  arc A10 (-67.22, -83.425) -> (-65.22, -85.425) centre (-65.22, -83.425) ccw
  line L85 (-67.22, -83.425) -> (-67.22, -75.425)
  arc A11 (-65.22, -73.425) -> (-67.22, -75.425) centre (-65.22, -75.425) ccw
  circle A12 centre (-103.4, 5) radius 1.45
  circle A13 centre (-103.4, -104.18) radius 1.45
  circle A14 centre (5, 5) radius 1.45
  circle A15 centre (5, -104.18) radius 1.45
  line L86 (-38, -98.9816) -> (-74.0181, -98.9816)
  line L87 (-74.0181, -98.9816) -> (-74.0181, -86)
  line L88 (-74.0181, -86) -> (-38, -86)
  line L89 (-38, -86) -> (-38, -98.9816)
  circle A16 centre (-44, -92.5) radius 5.5
  circle A17 centre (-44, -92.5) radius 5
  circle A18 centre (-44, -92.5) radius 4.5
  circle A19 centre (-44, -92.5) radius 4
  circle A20 centre (-44, -92.5) radius 3.5
  circle A21 centre (-44, -92.5) radius 3
  circle A22 centre (-44, -92.5) radius 2.5
  circle A23 centre (-44, -92.5) radius 2
  circle A24 centre (-44, -92.5) radius 1.5
  line L90 (-39.5, -88.5) -> (-48, -97)
  line L91 (-40, -88) -> (-48.5, -96.5)
  line L92 (-48.5, -96.5) -> (-48, -97)
  line L93 (-40, -88) -> (-39.5, -88.5)
  line L94 (-39.5, -97.5) -> (-48.5, -88.5)
  line L95 (-48.5, -88.5) -> (-48, -88)
  line L96 (-48, -88) -> (-39, -97)
  line L97 (-39, -97) -> (-39.5, -97.5)
  circle A25 centre (-56, -92.5) radius 2
  circle A26 centre (-56, -92.5) radius 4
  line L98 (-51, -97) -> (-51.5, -97.5)
  circle A27 centre (-56, -92.5) radius 5.5
  line L99 (-60, -88) -> (-51, -97)
  line L100 (-60.5, -96.5) -> (-60, -97)
  circle A28 centre (-56, -92.5) radius 5
  circle A29 centre (-56, -92.5) radius 3.5
  line L101 (-60.5, -88.5) -> (-60, -88)
  line L102 (-51.5, -97.5) -> (-60.5, -88.5)
  line L103 (-52, -88) -> (-60.5, -96.5)
  line L104 (-52, -88) -> (-51.5, -88.5)
  circle A30 centre (-56, -92.5) radius 1.5
  line L105 (-51.5, -88.5) -> (-60, -97)
  circle A31 centre (-56, -92.5) radius 3
  circle A32 centre (-56, -92.5) radius 4.5
  circle A33 centre (-56, -92.5) radius 2.5
  circle A34 centre (-68, -92.5) radius 2
  circle A35 centre (-68, -92.5) radius 4
  line L106 (-63, -97) -> (-63.5, -97.5)
  circle A36 centre (-68, -92.5) radius 5.5
  line L107 (-72, -88) -> (-63, -97)
  line L108 (-72.5, -96.5) -> (-72, -97)
  circle A37 centre (-68, -92.5) radius 5
  circle A38 centre (-68, -92.5) radius 3.5
  line L109 (-72.5, -88.5) -> (-72, -88)
  line L110 (-63.5, -97.5) -> (-72.5, -88.5)
  line L111 (-64, -88) -> (-72.5, -96.5)
  line L112 (-64, -88) -> (-63.5, -88.5)
  circle A39 centre (-68, -92.5) radius 1.5
  line L113 (-63.5, -88.5) -> (-72, -97)
  circle A40 centre (-68, -92.5) radius 3
  circle A41 centre (-68, -92.5) radius 4.5
  circle A42 centre (-68, -92.5) radius 2.5
  line L114 (-38, -94) -> (-74.0181, -94)
  line L115 (-74.0181, -94) -> (-74.0181, -91.0875)
  line L116 (-74.0181, -91.0875) -> (-38, -91.0875)
  line L117 (-38, -91.0875) -> (-38, -94)
  dimension "d86" = 11
  dimension "d87" = 10
  dimension "d88" = 9
  dimension "d89" = 8
  dimension "d90" = 7
  dimension "d91" = 6
  dimension "d92" = 5
  dimension "d93" = 4
  dimension "d94" = 3
  dimension "d95" = 11
  dimension "d96" = 10
  dimension "d97" = 9
  dimension "d98" = 8
  dimension "d99" = 7
  dimension "d100" = 6
  dimension "d101" = 5
  dimension "d102" = 4
  dimension "d103" = 3
  dimension "d104" = 11
  dimension "d105" = 10
  dimension "d106" = 9
  dimension "d107" = 8
  dimension "d108" = 7
  dimension "d109" = 6
  dimension "d110" = 5
  dimension "d111" = 4
  dimension "d112" = 3
  constraint horizontal L86
  constraint vertical L87
  constraint horizontal L88
  constraint vertical L89
  constraint concentric A16 A17
  constraint concentric A16 A18
  constraint concentric A16 A19
  constraint concentric A18 A20
  constraint concentric A17 A21
  constraint concentric A17 A22
  constraint concentric A17 A23
  constraint concentric A16 A24
  constraint perpendicular L90 L92
  constraint perpendicular L90 L93
  constraint perpendicular L94 L95
  constraint perpendicular L95 L96
  constraint perpendicular L94 L97
  constraint concentric A27 A28
  constraint concentric A27 A32
  constraint concentric A26 A27
  constraint concentric A29 A32
  constraint concentric A28 A31
  constraint concentric A28 A33
  constraint concentric A25 A28
  constraint concentric A27 A30
  constraint perpendicular L100 L105
  constraint perpendicular L104 L105
  constraint perpendicular L101 L102
  constraint perpendicular L99 L101
  constraint perpendicular L98 L102
  constraint concentric A36 A37
  constraint concentric A36 A41
  constraint concentric A35 A36
  constraint concentric A38 A41
  constraint concentric A37 A40
  constraint concentric A37 A42
  constraint concentric A34 A37
  constraint concentric A36 A39
  constraint perpendicular L108 L113
  constraint perpendicular L112 L113
  constraint perpendicular L109 L110
  constraint perpendicular L107 L109
  constraint perpendicular L106 L110
  constraint horizontal L114
  constraint vertical L115
  constraint horizontal L116
  constraint vertical L117
  constraint coincident L87 L115.end
  constraint coincident L89 L114.start
  measures "d86" diameter of A16
  measures "d87" diameter of A17
  measures "d88" diameter of A18
  measures "d89" diameter of A19
  measures "d90" diameter of A20
  measures "d91" diameter of A21
  measures "d92" diameter of A22
  measures "d93" diameter of A23
  measures "d94" diameter of A24
  measures "d95" diameter of A27
  measures "d96" diameter of A28
  measures "d97" diameter of A32
  measures "d98" diameter of A26
  measures "d99" diameter of A29
  measures "d100" diameter of A31
  measures "d101" diameter of A33
  measures "d102" diameter of A25
  measures "d103" diameter of A30
  measures "d104" diameter of A36
  measures "d105" diameter of A37
  measures "d106" diameter of A41
  measures "d107" diameter of A35
  measures "d108" diameter of A38
  measures "d109" diameter of A40
  measures "d110" diameter of A42
  measures "d111" diameter of A34
  measures "d112" diameter of A39
extrude "Extrude10" cut sketch "Sketch10" against normal blind 5 contours A16 A17 L96 L114 | A36 A37 L111 L114 | A16 A17 L90 L116 | A36 A37 L110 L116 | A16 A17 L90 L94 | A18 A19 L96 L114 | A36 A37 L110 L113 | A35 L111 A41 L114 | A16 A17 L91 L96 | A18 A19 L90 L116 | A36 L107 A37 L111 | A35 L110 A41 L116 | A16 A17 L91 L114 | A18 A19 L90 L94 | A20 A21 L96 L114 | A36 L107 A37 L114 | A35 L110 L113 A41 | A38 L111 A40 L114 | A16 A17 L94 L116 | A18 A19 L91 L96 | A20 A21 L90 L116 | A36 A37 L113 L116 | A35 L107 L111 A41 | A38 L110 A40 L116 | A27 L99 A28 L114 | A18 A19 L91 L114 | A20 A21 L90 L94 | A27 A28 L103 L114 | A35 L107 A41 L114 | A38 L110 L113 A40 | A27 A28 L105 L116 | A18 A19 L94 L116 | A20 A21 L91 L96 | A22 L90 L116 | A22 A23 L90 L94 | A27 A28 L102 L116 | A35 L113 A41 L116 | L107 A38 L111 A40 | L110 A42 L116 | A34 L110 L113 A42 | A27 A28 L102 L105 | A26 L99 A32 L114 | A20 A21 L91 L114 | A26 L103 A32 L114 | L107 A38 A40 L114 | A27 L99 A28 L103 | A26 L105 A32 L116 | A20 A21 L94 L116 | A22 A23 L91 L96 | A26 L102 A32 L116 | A38 L113 A40 L116 | A34 L107 L111 A42 | A26 L102 L105 A32 | L99 A29 A31 L114 | A22 L94 L116 | A29 L103 A31 L114 | A26 L99 L103 A32 | A29 L105 A31 L116 | A24 L116 | A29 L102 A31 L116 | L113 A42 L116 | A39 L116 | A29 L102 L105 A31 | L99 A29 L103 A31 | L105 A33 L116 | A25 L102 L105 A33 | L102 A33 L116 | A25 L99 L103 A33 | A30 L116 bodies 2
sketch "Sketch11" plane through (0, 0, 0) normal (0, -1, 0) x (1, 0, 0)
  arc A0 (108.4, 5) -> (103.4, 10) centre (103.4, 5) ccw
  line L0 (103.4, 10) -> (-5, 10)
  arc A1 (-5, 10) -> (-10, 5) centre (-5, 5) ccw
  line L1 (-10, 5) -> (-10, -104.18)
  arc A2 (-10, -104.18) -> (-5, -109.18) centre (-5, -104.18) ccw
  line L2 (-5, -109.18) -> (103.4, -109.18)
  arc A3 (103.4, -109.18) -> (108.4, -104.18) centre (103.4, -104.18) ccw
  line L3 (108.4, -104.18) -> (108.4, 5)
  circle A4 centre (-5, -104.18) radius 1.45
  circle A5 centre (103.4, 5) radius 1.45
  circle A6 centre (103.4, -104.18) radius 1.45
  circle A7 centre (-5, 5) radius 1.45
  line L4 (75, -75) -> (25, -75)
  line L5 (25, -75) -> (25, -25)
  line L6 (25, -25) -> (75, -25)
  line L7 (75, -25) -> (75, -75)
  constraint horizontal L4
  constraint vertical L5
  constraint horizontal L6
  constraint vertical L7
extrude "Extrude11" cut sketch "Sketch11" against normal blind 3 contours L4 L5 L6 L7 bodies 1
chamfer "Chamfer1" distance 3 angle 45 1 edges at (50, 0, -25) on bodies 1
chamfer "Chamfer2" distance 3 angle 45 1 edges at (50, 0, -75) on bodies 1
chamfer "Chamfer3" distance 3 angle 45 1 edges at (75, 0, -50) on bodies 1
extrude "Extrude12" add 1 faces at (1.6667, 0, -40.3935) along direction (0, -1, 0) blind 3 separate body on bodies 1 makes body 3
chamfer "Chamfer4" distance 3 angle 45 1 edges at (78, -3, -50) on bodies 3
chamfer "Chamfer5" distance 3 angle 45 1 edges at (53, -3, -78) on bodies 3
chamfer "Chamfer6" distance 3 angle 45 1 edges at (53, -3, -22) on bodies 3
hole "Hole1" at (12.5086, -3, -64.3972) direction (0, 1, 0) diameter 20 depth 7 tip angle 118 bodies 1 3
fillet "Fillet17" radius 2 1 edges at (16.1248, -3, -55.0739) on bodies 3
chamfer "Chamfer7" distance 1 angle 45 1 edges at (8.8925, 2.9461, -55.0739) on bodies 1
hole "Hole2" at (12.3349, 2.9461, -38.8752) direction (0, -1, 0) diameter 20 depth 15 tip angle 118 bodies 1 3
fillet "Fillet18" radius 2 1 edges at (8.7188, -3, -48.1985) on bodies 3
chamfer "Chamfer8" distance 1 angle 45 1 edges at (15.9511, 2.9461, -48.1985) on bodies 1